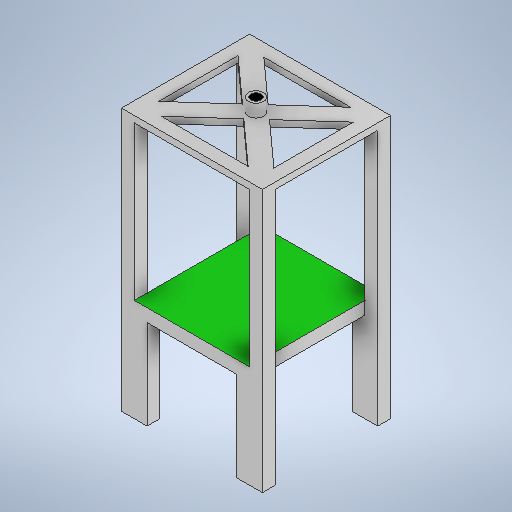
# Autodesk Inventor part: Soporte_Corte
Saved by Autodesk Inventor 2025.2 (Build 292293000, 293)
## iProperties
Created: 2025-02-05
Part Number: Soporte_Corte
Material: Generic
Document SubType Name: Modeling
Designer: Proyectos
Density: 1 g/cm^3
Appearance: Default
Author: Proyectos
Autodesk Inventor part; units mm, degrees
ref_plane "YZ Plane" through (0, 0, 0) normal (1, 0, 0) x (0, 1, 0)
ref_plane "XZ Plane" through (0, 0, 0) normal (0, 1, 0) x (-1, 0, 0)
ref_plane "XY Plane" through (0, 0, 0) normal (0, 0, 1) x (1, 0, 0)
sketch "Sketch2" plane through (0, 0, 0) normal (0, 1, 0) x (-1, 0, 0)
  line L0 (0, 0) -> (900, 0)
  line L1 (900, 0) -> (900, -1000)
  line L2 (900, -1000) -> (0, -1000)
  line L3 (0, -1000) -> (0, 0)
  dimension "d0" = 900
  dimension "d1" = 1000
  constraints: 8 end point, 2 parallel, 1 horizontal, 1 perpendicular
  measures "d0" distance of L1.end L2.end
  measures "d1" distance of L2.end L0.start
extrude "Extrusion1" add sketch "Sketch2" along normal blind 800
sketch "Sketch3" plane through (-900, 0, 0) normal (0, 0, 1) x (1, 0, 0)
  line L0 (900, 0) -> (0, 0) projected
  line L1 (0, 0) -> (100, 0)
  line L2 (900, 0) -> (900, 800) projected
  line L3 (900, 0) -> (800, 0)
  line L4 (800, 0) -> (100, 0)
  line L5 (100, 0) -> (100, 700)
  line L6 (100, 700) -> (800, 700)
  line L7 (800, 700) -> (800, 0)
  dimension "d4" = 100
  dimension "d5" = 100
  dimension "d6" = 700
  constraints: 12 end point, 2 parallel, 2 point on line, 1 horizontal, 1 perpendicular
  measures "d4" distance of L0.end L1.end
  measures "d5" distance of L0.start L3.end
  measures "d6" distance of L4.end L5.end
extrude "Extrusion2" cut sketch "Sketch3" against normal through all
sketch "Sketch4" plane through (0, 0, 0) normal (1, 0, 0) x (0, 0, -1)
  line L0 (0, 0) -> (100, 0)
  line L1 (1000, 0) -> (0, 0) projected
  line L2 (1000, 0) -> (900, 0)
  line L3 (0, 700) -> (1000, 700) projected
  line L4 (900, 0) -> (100, 0)
  line L5 (100, 0) -> (100, 700)
  line L6 (100, 700) -> (900, 700)
  line L7 (900, 700) -> (900, 0)
  dimension "d9" = 100
  dimension "d10" = 100
  constraints: 12 end point, 3 point on line, 2 parallel, 1 horizontal, 1 perpendicular
  measures "d9" distance of L0.start L0.end
  measures "d10" distance of L1.start L2.end
extrude "Extrusion3" cut sketch "Sketch4" against normal through all
sketch "Sketch5" plane through (0, 0, 0) normal (0, -1, 0) x (1, 0, 0)
  line L0 (-900, -100) -> (-800, -100) projected
  line L1 (-800, -100) -> (-800, 0) projected
  line L2 (-900, 0) -> (-800, 0) projected
  line L3 (-900, -100) -> (-900, 0) projected
  line L4 (-800, -900) -> (-900, -900) projected
  line L5 (-900, -1000) -> (-900, -900) projected
  line L6 (-800, -1000) -> (-900, -1000) projected
  line L7 (-800, -1000) -> (-800, -900) projected
  line L8 (0, -900) -> (-100, -900) projected
  line L9 (-100, -900) -> (-100, -1000) projected
  line L10 (0, -1000) -> (-100, -1000) projected
  line L11 (0, -900) -> (0, -1000) projected
  line L12 (-100, -100) -> (0, -100) projected
  line L13 (0, 0) -> (0, -100) projected
  line L14 (-100, 0) -> (0, 0) projected
  line L15 (-100, 0) -> (-100, -100) projected
  line L16 (0, -100) -> (-100, -100) projected
  line L17 (0, -100) -> (100, -100)
  line L18 (100, -100) -> (100, 0)
  line L19 (100, 0) -> (0, 0)
  line L20 (0, 0) -> (0, -100)
  line L21 (0, -900) -> (100, -900)
  line L22 (100, -900) -> (100, -1000)
  line L23 (100, -1000) -> (0, -1000)
  line L24 (0, -1000) -> (0, -900)
  line L25 (-900, -1000) -> (-1000, -1000)
  line L26 (-1000, -1000) -> (-1000, -900)
  line L27 (-1000, -900) -> (-900, -900)
  line L28 (-900, -900) -> (-900, -1000)
  line L29 (-900, 0) -> (-1000, 0)
  line L30 (-1000, 0) -> (-1000, -100)
  line L31 (-1000, -100) -> (-900, -100)
  line L32 (-900, -100) -> (-900, 0)
  dimension "d13" = 100
  dimension "d14" = 100
  constraints: 32 end point, 8 parallel, 4 horizontal, 4 perpendicular, 2 point on line
  measures "d13" distance of L19.end L18.end
  measures "d14" distance of L26.end L27.end
extrude "Extrusion4" add sketch "Sketch5" against normal blind 2000 contours L31 L30 L29 L3 | L5 L25 L26 L27 | L21 L22 L23 L11 | L13 L19 L18 L17
sketch "Sketch6" plane through (0, 2000, 0) normal (0, 1, 0) x (1, 0, 0)
  line L0 (-1000, 1000) -> (-1000, 900) projected
  line L1 (100, 0) -> (100, 100) projected
  line L2 (-1000, 0) -> (-900, 0) projected
  line L3 (100, 1000) -> (100, 900) projected
  line L4 (100, 1000) -> (-100, 1000) projected
  line L5 (-1000, 0) -> (100, 0)
  line L6 (100, 0) -> (100, 1000)
  line L7 (100, 1000) -> (-1000, 1000)
  line L8 (-1000, 1000) -> (-1000, 0)
  line L9 (-1000, 0) -> (100, 1000) construction
  line L10 (100, 0) -> (-1000, 1000) construction
  line L11 (-1000, 1000) -> (-900, 1000)
  line L12 (-900, 1000) -> (-900, 0)
  line L13 (-900, 0) -> (-1000, 0)
  line L14 (-1000, 0) -> (-1000, 1000)
  line L15 (100, 0) -> (-1000, 0)
  line L16 (-1000, 0) -> (-1000, 100)
  line L17 (-1000, 100) -> (100, 100)
  line L18 (100, 100) -> (100, 0)
  line L19 (0, 1000) -> (100, 1000)
  line L20 (100, 1000) -> (100, 0)
  line L21 (100, 0) -> (0, 0)
  line L22 (0, 0) -> (0, 1000)
  line L23 (-1000, 900) -> (100, 900)
  line L24 (100, 900) -> (100, 1000)
  line L25 (100, 1000) -> (-1000, 1000)
  line L26 (-1000, 1000) -> (-1000, 900)
  line L27 (-1000, 900) -> (0, 0)
  line L28 (-900, 1000) -> (100, 100)
  line L29 (-1000, 100) -> (0, 1000)
  line L30 (-900, 0) -> (100, 900)
  point P0 (-450, 500)
  point P1 (-788.8889, 100)
  point P2 (-450, 405)
  point P3 (-111.1111, 100)
  point P4 (-100, 1000)
  point P5 (-111.1111, 900)
  point P6 (-450, 595)
  point P7 (-788.8889, 900)
  point P8 (0, 810)
  point P9 (0, 190)
  point P10 (-344.4444, 500)
  point P11 (-900, 190)
  point P12 (-900, 810)
  point P13 (-555.5556, 500)
  constraints: 52 end point, 12 parallel, 5 horizontal, 5 perpendicular, 2 midpoint, 2 point on line
extrude "Extrusion5" add sketch "Sketch6" along normal blind 50 contours L7 L12 L23 L0 | L27 L12 L29 L8 | L23 L12 L27 | L28 L23 L12 | L7 L4 L29 L23 L28 | L17 L12 L2 L8 | L29 L12 L17 | L23 L28 L29 L27 L12 | L17 L30 L12 | L12 L29 L27 L30 L17 | L29 L28 L30 L27 | L4 L3 L23 L22 | L22 L23 L29 | L23 L22 L30 L28 L29 | L30 L17 L27 L5 | L30 L28 L22 L17 L27 | L23 L30 L22 | L22 L17 L1 L5 | L27 L17 L22 | L6 L28 L22 L30 | L28 L17 L22
sketch "Sketch7" plane through (0, 2050, 0) normal (0, 1, 0) x (1, 0, 0)
  line L0 (-555.5556, 500) -> (-900, 190) projected
  line L1 (0, 190) -> (-344.4444, 500) projected
  line L2 (-555.5556, 500) -> (-344.4444, 500)
  line L3 (-111.1111, 900) -> (-450, 595) projected
  line L4 (-450, 405) -> (-111.1111, 100) projected
  line L5 (-450, 595) -> (-450, 405)
  circle A0 centre (-450, 500) radius 50
  circle A1 centre (-450, 500) radius 40
  point P0 (0, 0)
  dimension "d19" = 100
  dimension "d20" = 80
  constraints: 4 end point, 2 centre point, 1 coincident, 1 horizontal, 1 midpoint, 1 vertical
  measures "d19" diameter of A0
  measures "d20" diameter of A1
extrude "Extrusion6" cut sketch "Sketch7" against normal blind 200 contours A1 L5 L2 | L2 L5 A1 | L5 A1 L2 | L2 A1 L5
sketch "Sketch8" plane through (0, 2050, 0) normal (0, 1, 0) x (1, 0, 0)
  circle A0 centre (-450, 500) radius 40 projected
  circle A1 centre (-450, 500) radius 60
  point P0 (0, 0)
  dimension "d23" = 120
  constraints: 1 centre point, 1 coincident
  measures "d23" diameter of A1
extrude "Extrusion7" add sketch "Sketch8" along normal blind 100
body "Solid1"
